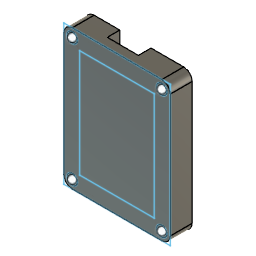
laya's hackpad (Autodesk Fusion 360 design; units mm, degrees)
part number: 2026-02-03-13-53-59-911
Autodesk Fusion 360 part; units mm, degrees
sketch "Sketch1" plane through (0, 0, 0) normal (0, 1, 0) x (1, 0, 0)
  line L0 (-44.6765, -46.7839) -> (-0.4215, -46.7839)
  line L1 (-0.4215, -46.7839) -> (-0.4215, 17.2161)
  line L2 (-0.4215, 17.2161) -> (-44.6765, 17.2161)
  line L3 (-44.6765, 17.2161) -> (-44.6765, -46.7839)
  line L4 (-54.1765, -56.2839) -> (9.0449, -56.2839)
  line L5 (9.0449, -56.2839) -> (9.0449, 26.7161)
  line L6 (9.0449, 26.7161) -> (-54.1765, 26.7161)
  line L7 (-54.1765, 26.7161) -> (-54.1765, -56.2839)
  circle A0 centre (-49.1765, -51.2839) radius 1.7
  circle A1 centre (-49.1765, 21.7161) radius 1.7
  circle A2 centre (4.0449, 21.7161) radius 1.7
  circle A3 centre (4.0449, -51.2839) radius 1.7
  circle A4 centre (-49.1765, -51.2839) radius 3
  circle A5 centre (4.0449, -51.2839) radius 3
  circle A6 centre (4.0449, 21.7161) radius 3
  circle A7 centre (-49.1765, 21.7161) radius 3
  dimension "d1" = 64
  dimension "d2" = 83
  dimension "d3" = 9.5
  dimension "d4" = 9.5
  dimension "d5" = 3.4
  dimension "d6" = 5
  dimension "d7" = 5
  dimension "d8" = 3.4
  dimension "d9" = 63.2214
  dimension "d10" = 5
  dimension "d11" = 5
  dimension "d12" = 3.4
  dimension "d13" = 5
  dimension "d14" = 5
  dimension "d15" = 3.4
  dimension "d16" = 5
  dimension "d17" = 5
  dimension "d18" = 6
  dimension "d19" = 6
  dimension "d20" = 6
  dimension "d21" = 6
  constraint horizontal L0
  constraint vertical L1
  constraint horizontal L2
  constraint vertical L3
  constraint horizontal L4
  constraint vertical L5
  constraint horizontal L6
  constraint vertical L7
  constraint concentric A0 A4
  constraint concentric A3 A5
  constraint concentric A2 A6
  constraint concentric A1 A7
  measures "d1" distance of L0.start L2.end
  measures "d2" distance of L4.start L6.end
  measures "d3" distance of L0 L4
  measures "d4" distance of L3 L7
  measures "d5" diameter of A0
  measures "d6" distance of L7 A0.centre
  measures "d7" distance of L4 A0.centre
  measures "d8" diameter of A1
  measures "d9" distance of L5.end L6.end
  measures "d10" distance of L6 A1.centre
  measures "d11" distance of L7 A1.centre
  measures "d12" diameter of A2
  measures "d13" distance of L5 A2.centre
  measures "d14" distance of L6 A2.centre
  measures "d15" diameter of A3
  measures "d16" distance of L5 A3.centre
  measures "d17" distance of L4 A3.centre
  measures "d18" diameter of A4
  measures "d19" diameter of A5
  measures "d20" diameter of A6
  measures "d21" diameter of A7
extrude "Extrude1" add sketch "Sketch1" along normal blind 9.9 from surface at 3.1 contours A4 | A5 | A6 | A7 makes body 1 at (-51.5679, 9.7, 49.4724) makes body 2 at (7.0412, 9.7, -21.5666) makes body 3 at (7.0412, 9.7, 51.4334) makes body 4 at (-46.1802, 9.7, -21.5666)
extrude "Extrude2" add sketch "Sketch1" along normal blind 13 contours L4 L5 L6 L7 bodies 1 2 3 4
extrude "Extrude3" add sketch "Sketch1" along normal blind 3 contours L0 L1 L2 L3 bodies 1
sketch "Sketch2" plane through (0, 13, 0) normal (0, 1, 0) x (-1, 0, 0)
  circle A0 centre (49.1765, 51.2839) radius 1.7
  circle A1 centre (49.1765, -21.7161) radius 1.7
  line L0 (44.6765, 46.7839) -> (44.6765, -17.2161)
  line L1 (44.6765, -17.2161) -> (0.4215, -17.2161)
  line L2 (0.4215, -17.2161) -> (0.4215, 46.7839)
  line L3 (0.4215, 46.7839) -> (44.6765, 46.7839)
  line L4 (54.1765, -26.7161) -> (54.1765, 56.2839)
  line L5 (54.1765, 56.2839) -> (-9.0449, 56.2839)
  line L6 (-9.0449, 56.2839) -> (-9.0449, -26.7161)
  line L7 (-9.0449, -26.7161) -> (54.1765, -26.7161)
  circle A2 centre (-4.0449, -21.7161) radius 1.7
  circle A3 centre (-4.0449, 51.2839) radius 1.7
  line L8 (15.3881, 56.2839) -> (33.8881, 56.2839)
  line L9 (33.8881, 56.2839) -> (33.8881, 46.7839)
  line L10 (33.8881, 46.7839) -> (15.3881, 46.7839)
  line L11 (15.3881, 46.7839) -> (15.3881, 56.2839)
  line L12 (-9.0449, 56.2839) -> (-9.0449, -26.7161)
  dimension "d29" = 18.5
  dimension "d30" = 24.433
  constraint horizontal L8
  constraint vertical L9
  constraint horizontal L10
  constraint vertical L11
  constraint coincident L3 L9.end
  constraint coincident L5 L8.start
  measures "d29" distance of L9 L11
  measures "d30" distance of L11 L12
extrude "Extrude4" cut sketch "Sketch2" against normal blind 7.5 contours L3 L5 L8 L9 L10 L11 bodies 1
fillet "Fillet1" radius 5 1 edges at (9.0449, 6.5, 56.2839) on bodies 1
fillet "Fillet2" radius 5 1 edges at (-54.1765, 6.5, 56.2839) on bodies 1
fillet "Fillet3" radius 5 1 edges at (-54.1765, 6.5, -26.7161) on bodies 1
fillet "Fillet4" radius 5 1 edges at (9.0449, 6.5, -26.7161) on bodies 1
